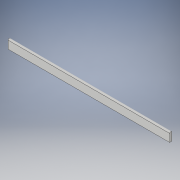
# Autodesk Inventor part: belka
Saved by Autodesk Inventor 2019 (Build 230136000, 136)
## iProperties
Created: 2020-01-12
Part Number: belka
Material: Ogólny
Document SubType Name: Modeling
Designer: Karolina
Density: 1 g/cm^3
Appearance: Domyślna
Author: Karolina
Autodesk Inventor part; units mm, degrees
ref_plane "YZ Plane" through (0, 0, 0) normal (1, 0, 0) x (0, 1, 0)
ref_plane "XZ Plane" through (0, 0, 0) normal (0, 1, 0) x (-1, 0, 0)
ref_plane "XY Plane" through (0, 0, 0) normal (0, 0, 1) x (1, 0, 0)
sketch "Szkic1" plane through (0, 0, 0) normal (0, 0, 1) x (1, 0, 0)
  line L0 (0, -0.8) -> (0, 4.8) construction
  line L1 (-14.48, 0) -> (86.88, 0) construction
  line L2 (0, 0) -> (72.4, 0)
  line L3 (72.4, 0) -> (72.4, 4)
  line L4 (72.4, 4) -> (0, 4)
  line L5 (0, 4) -> (0, 0)
  dimension "d0" = 4
  dimension "d1" = 72.4
  constraints: 8 end point, 2 parallel, 1 horizontal, 1 perpendicular
  measures "d0" distance of L2.end L3.end
  measures "d1" distance of L3.end L4.end
extrude "Wyciągnięcie proste1" add sketch "Szkic1" along normal blind 1
fillet "Zaokrąglenie1" radius 0.5 2 edges at (36.2, 4, 1) (36.2, 4, 0)
